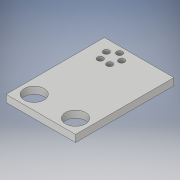
# Autodesk Inventor part: Side Peices
Saved by Autodesk Inventor 2019 (Build 230136000, 136)
## iProperties
Created: 2018-12-01
Part Number: Side Peices
Material: Generic
Document SubType Name: Modeling
Designer: Ashley
Density: 1 g/cm^3
Appearance: Default
Author: Ashley
Autodesk Inventor part; units mm, degrees
ref_plane "YZ Plane" through (0, 0, 0) normal (1, 0, 0) x (0, 1, 0)
ref_plane "XZ Plane" through (0, 0, 0) normal (0, 1, 0) x (-1, 0, 0)
ref_plane "XY Plane" through (0, 0, 0) normal (0, 0, 1) x (1, 0, 0)
sketch "Sketch1" plane through (0, 0, 0) normal (0, 1, 0) x (-1, 0, 0)
  line L0 (-27.4, -50) -> (22, -50)
  line L1 (22, -50) -> (22, 20)
  line L2 (22, 20) -> (-27.4, 20)
  line L3 (-27.4, 20) -> (-27.4, -50)
  line L4 (2, 20) -> (-2, 20)
  circle A0 centre (12, 10) radius 7.1
  circle A1 centre (-17.4, 10) radius 7.1
  circle A2 centre (7, -45.7) radius 2.1
  circle A3 centre (12.421, -41.7614) radius 2.1
  circle A4 centre (10.3504, -35.3886) radius 2.1
  circle A5 centre (3.6496, -35.3886) radius 2.1
  circle A6 centre (1.579, -41.7614) radius 2.1
  circle A7 centre (12, 10) radius 14.625 construction
  circle A8 centre (-17.4, 10) radius 14.625 construction
  point P0 (0, 0)
  point P1 (7, -40)
  dimension "d1" = 70
  dimension "d8" = 10
  dimension "d9" = 14.2
  dimension "d10" = 14.2
  dimension "d11" = 10
  dimension "d13" = 10
  dimension "d16" = 4.2
  dimension "d17" = 5.7
  dimension "d20" = 360
  dimension "d22" = 10
  dimension "d27" = 29.25
  dimension "d28" = 29.25
  dimension "d29" = 29.4
  dimension "d30" = 10
  dimension "d31" = 15
  constraints: 10 end point, 9 centre point, 2 coincident, 2 horizontal, 2 parallel, 1 perpendicular, 1 point on line, 12 other
  measures "d1" distance between parallel lines of L0 L2
  measures "d8" distance from line of A0.centre L1
  measures "d9" diameter of A0
  measures "d10" diameter of A1
  measures "d11" distance from line of L2 A1.centre
  measures "d13" distance from line of L2 A0.centre
  measures "d16" diameter of A2
  measures "d17" distance of point (7, -40) A2.centre
  measures "d22" distance from line of L0 point (7, -40)
  measures "d27" diameter of A7
  measures "d28" diameter of A8
  measures "d29" distance of A1.centre A0.centre
  measures "d30" distance from line of L3 A1.centre
  measures "d31" distance from line of L1 point (7, -40)
extrude "Extrusion3" add sketch "Sketch1" along normal blind 5
body "Solid3"
